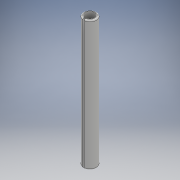
# Autodesk Inventor part: 5x65彈簧銷
Saved by Autodesk Inventor 2018 (Build 220112000, 112)
## iProperties
Created: 2024-12-04
Part Number: 5x65彈簧銷
Material: 一般
Document SubType Name: Modeling
Designer: User
Density: 1 g/cm^3
Appearance: 預設
Author: User
Autodesk Inventor part; units mm, degrees
ref_plane "YZ Plane" through (0, 0, 0) normal (1, 0, 0) x (0, 1, 0)
ref_plane "XZ Plane" through (0, 0, 0) normal (0, 1, 0) x (-1, 0, 0)
ref_plane "XY Plane" through (0, 0, 0) normal (0, 0, 1) x (1, 0, 0)
sketch "草圖1" plane through (0, 0, 0) normal (0, 0, 1) x (1, 0, 0)
  arc A0 (0.3, -2.4819) -> (-0.3, -2.4819) centre (0, 0) ccw
  arc A1 (0.3, -1.7241) -> (-0.3, -1.7241) centre (0, 0) ccw
  line L0 (0.3, -1.7241) -> (0.3, -2.4819)
  line L1 (-0.3, -2.4819) -> (-0.3, -1.7241)
  dimension "d0" = 5
  dimension "d1" = 3.5
  dimension "d2" = 0.3
  dimension "d3" = 0.6
  constraints: 4 end point, 4 point on circle, 2 centre point, 2 coincident, 1 parallel
  measures "d0" diameter of A0
  measures "d1" diameter of A1
  measures "d2" distance from line of point (0, 0) L1
  measures "d3" distance between parallel lines of L1 L0
extrude "擠出1" add sketch "草圖1" along normal blind 50
fillet "圓角1" radius 0.5 2 edges at (0, 2.5, 50) (0, 2.5, 0)
